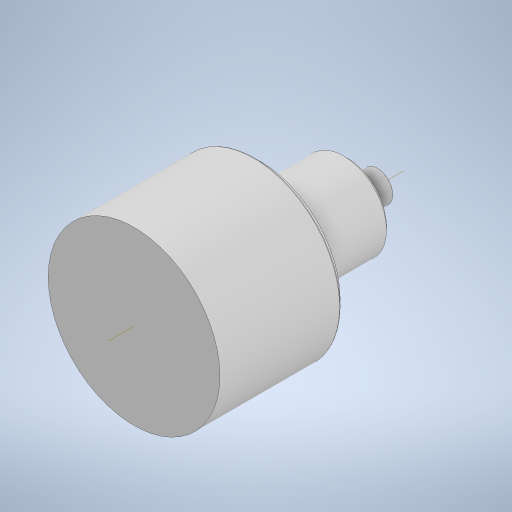
# Autodesk Inventor part: eje (bolt)
Saved by Autodesk Inventor 2024.3 (Build 283343000, 343)
## iProperties
Created: 2025-07-04
Part Number: eje (bolt)
Material: Genérico
Document SubType Name: Modeling
Designer: Daniel Rodriguez
Density: 1 g/cm^3
Appearance: Valor por defecto
Author: Daniel Rodriguez
Autodesk Inventor part; units mm, degrees
ref_plane "YZ Plane" through (0, 0, 0) normal (1, 0, 0) x (0, 1, 0)
ref_plane "XZ Plane" through (0, 0, 0) normal (0, 1, 0) x (-1, 0, 0)
ref_plane "XY Plane" through (0, 0, 0) normal (0, 0, 1) x (1, 0, 0)
sketch "Boceto1" plane through (0, 0, 0) normal (0, 0, 1) x (1, 0, 0)
  circle A0 centre (0, 0) radius 125
  dimension "d0" = 250
  constraints: 1 centre point, 1 coincident
  measures "d0" diameter of A0
extrude "Extrusión1" add sketch "Boceto1" against normal blind 185
sketch "Boceto2" plane through (0, 0, -185) normal (0, 0, -1) x (-1, 0, 0)
  circle A0 centre (0, 0) radius 62.5
  dimension "d3" = 125
  constraints: 1 centre point, 1 coincident
  measures "d3" diameter of A0
extrude "Extrusión2" add sketch "Boceto2" along normal blind 125
sketch "Boceto3" plane through (0, 0, -310) normal (0, 0, -1) x (-1, 0, 0)
  circle A0 centre (0, 0) radius 22.5
  dimension "d6" = 45
  constraints: 1 centre point, 1 coincident
  measures "d6" diameter of A0
extrude "Extrusión3" add sketch "Boceto3" along normal blind 45
chamfer "Chaflán1" distance 10 angle 45 1 edges at (-125, 0, -185)
fillet "Empalme1" radius 2 2 edges at (-125, 0, -175) (-115, 0, -185)
fillet "Empalme de cara1" radius 30 1 edges at (62.5, 0, -185)
chamfer "Chaflán2" distance 5 angle 45 1 edges at (62.5, 0, -310)
fillet "Empalme2" radius 1 1 edges at (22.5, 0, -355)
fillet "Empalme de cara2" radius 4 1 edges at (22.5, 0, -310)
equation "\"d3\" = 0.5 * d0"
